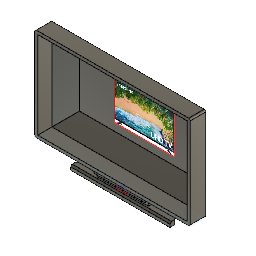
samsung tv v1 v1 (Autodesk Fusion 360 design; units mm, degrees)
Autodesk Fusion 360 part; units mm, degrees
sketch "Sketch1" plane through (0, 0, 0) normal (0, 1, 0) x (1, 0, 0)
  line L0 (0, 0) -> (100, 0)
  line L1 (100, 0) -> (100, -60)
  line L2 (100, -60) -> (0, -60)
  line L3 (0, -60) -> (0, 0)
  constraint horizontal L0
  constraint vertical L1
  constraint horizontal L2
  constraint vertical L3
  constraint coincident L0.start L3.end
extrude "Extrude1" add sketch "Sketch1" along normal blind 20
chamfer "Chamfer1" distance 10 angle 45 1 edges at (50, 20, 60)
chamfer "Chamfer2" distance 10 angle 45 1 edges at (50, 20, 0)
chamfer "Chamfer3" distance 10 angle 45 1 edges at (0, 20, 30)
chamfer "Chamfer4" distance 10 angle 45 1 edges at (100, 20, 30)
shell "Shell1" thickness 2 removed faces 1 at (33.3333, 0, 20)
sketch "Sketch2" plane through (0, 0, 0) normal (0, 0, -1) x (1, 0, 0)
  line L0 (0, -10) -> (100, -10)
  line L1 (100, -10) -> (100, 0)
  line L2 (100, 0) -> (0, 0)
  line L3 (0, 0) -> (0, -10)
  line L4 (35.198, -6.5843) -> (68.0611, -6.5843)
  line L5 (68.0611, -6.5843) -> (68.0611, -3.0276)
  line L6 (68.0611, -3.0276) -> (35.198, -3.0276)
  line L7 (35.198, -3.0276) -> (35.198, -6.5843)
  constraint horizontal L4
  constraint vertical L5
  constraint horizontal L6
  constraint vertical L7
extrude "Extrude2" add sketch "Sketch2" along normal blind 5 contours L4 L5 L6 L7
sketch "Sketch3" plane through (0, 0, 0) normal (0, 0, -1) x (1, 0, 0)
  line L0 (35.198, -3.0276) -> (68.0611, -3.0276)
  line L1 (68.0611, -3.0276) -> (68.0611, -6.5843)
  line L2 (68.0611, -6.5843) -> (35.198, -6.5843)
  line L3 (35.198, -6.5843) -> (35.198, -3.0276)
  line L4 (0, -10) -> (100, -10)
  line L5 (100, -10) -> (100, 0)
  line L6 (100, 0) -> (0, 0)
  line L7 (0, 0) -> (0, -10)
fillet "Fillet1" radius 1 1 edges at (100, 5, 60)
fillet "Fillet2" radius 1 1 edges at (0, 5, 60)
fillet "Fillet3" radius 1 1 edges at (100, 5, 0)
fillet "Fillet4" radius 1 1 edges at (0, 5, 0)
sketch "Sketch4" plane through (0, 0, 0) normal (1, 0, 0) x (0, 1, 0)
sketch "Sketch5" plane through (0, 3.5858, -3.5858) normal (0, -0.707107, 0.707107) x (1, 0, 0)
  line L0 (98, 7.8995) -> (89.1716, 20.3848)
  line L1 (89.1716, 20.3848) -> (10.8284, 20.3848)
  line L2 (10.8284, 20.3848) -> (2, 7.8995)
  line L3 (2, 7.8995) -> (98, 7.8995)
  line L4 (27.7452, 0) -> (75.1178, 0)
  line L5 (75.1178, 0) -> (75.1178, -10)
  line L6 (75.1178, -10) -> (27.7452, -10)
  line L7 (27.7452, -10) -> (27.7452, 0)
  dimension "d15" = 10
  constraint horizontal L4
  constraint vertical L5
  constraint horizontal L6
  constraint vertical L7
  measures "d15" distance of L4.end L5.end
extrude "Extrude3" cut sketch "Sketch5" against normal blind 8 contours L4 L5 L6 L7
extrude "Extrude4" add 1 faces at (46.1524, 5.5281, -5) along direction (0, 0, -1) blind 2
sketch "Sketch6" plane through (0, 0, 0) normal (1, 0, 0) x (0, 1, 0)
  line L0 (3, -7) -> (7, -7)
  line L1 (7, -7) -> (7, -10)
  line L2 (7, -10) -> (3, -10)
  line L3 (3, -10) -> (3, -7)
  constraint horizontal L0
  constraint vertical L1
  constraint horizontal L2
  constraint vertical L3
extrude "Extrude5" add sketch "Sketch6" along normal blind 100
extrude "Extrude6" cut 1 faces at (0, 4.3333, -8) along direction (1, 0, 0) blind 20
extrude "Extrude7" cut 1 faces at (100, 4.3333, -8) along direction (-1, 0, 0) blind 16
chamfer "Chamfer5" distance 1 angle 45 1 edges at (52, 3, -7)
chamfer "Chamfer6" distance 1 angle 45 1 edges at (84, 7, -8.5)
chamfer "Chamfer7" distance 1 angle 45 1 edges at (20, 7, -8.5)
